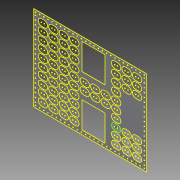
# Autodesk Inventor part: baseplate archive
Saved by Autodesk Inventor 2014 SP1 (Build 180222100, 222)
## iProperties
Created: 2014-01-05
Part Number: baseplate archive
Material: Aluminum 6061
Document SubType Name: Sheet Metal
Designer: Arpan
Density: 2.71 g/cm^3
Sheet Metal Rule: Default
Appearance: Aluminum - Flat
Mass: 756.379 g
Surface Area: 3765.41 cm^2
Volume: 279.107 cm^3
Author: Arpan
Autodesk Inventor part; units mm, degrees
(part 1 of 2)
ref_plane "YZ Plane" through (0, 0, 0) normal (1, 0, 0) x (0, 1, 0)
ref_plane "XZ Plane" through (0, 0, 0) normal (0, 1, 0) x (-1, 0, 0)
ref_plane "XY Plane" through (0, 0, 0) normal (0, 0, 1) x (1, 0, 0)
sketch "Sketch1" plane through (0, 0, 0) normal (0, 0, 1) x (1, 0, 0)
  line L0 (0, 0) -> (-685.8, 0)
  line L1 (-685.8, 0) -> (-685.8, 516.255)
  line L2 (-685.8, 516.255) -> (0, 516.255)
  line L3 (0, 516.255) -> (0, 0)
  dimension "d0" = 685.8
  dimension "d1" = 516.255
  measures "d0" distance of L1.end L2.end
  measures "d1" distance of L2.end L0.start
extrude "Plate1" add sketch "Sketch1" along normal blind 1.5875
sketch "Sketch4" plane through (0, 0, 1.5875) normal (0, 0, 1) x (1, 0, 0)
  circle A0 centre (-673.1, 503.555) radius 2.0828 projected
  circle A1 centre (-673.1, 12.7) radius 2.0828 projected
extrude "Cut3" cut sketch "Sketch4" against normal blind 1.5875
pattern_linear "Rectangular Pattern2" count 27 spacing 25.4 along (1, 0, 0) of "Cut3"
sketch "Sketch5" plane through (0, 0, 1.5875) normal (0, 0, 1) x (1, 0, 0)
  line L0 (-685.8, 516.255) -> (0, 516.255)
  line L1 (0, 516.255) -> (0, 0)
  line L2 (0, 0) -> (-685.8, 0)
  line L3 (-685.8, 0) -> (-685.8, 516.255)
  line L4 (-25.4, 490.855) -> (-660.4, 490.855)
  line L5 (-660.4, 490.855) -> (-660.4, 25.4)
  line L6 (-660.4, 25.4) -> (-25.4, 25.4)
  line L7 (-25.4, 25.4) -> (-25.4, 490.855)
  line L8 (-660.4, 490.855) -> (-596.9, 490.855)
  line L9 (-596.9, 490.855) -> (-596.9, 444.3095)
  line L10 (-596.9, 444.3095) -> (-660.4, 444.3095)
  line L11 (-660.4, 467.5822) -> (-596.9, 467.5822) construction
  line L12 (-637.1273, 444.3095) -> (-620.1728, 444.3095)
  line L13 (-620.1728, 490.855) -> (-637.1273, 490.855)
  arc A0 (-637.1273, 490.855) -> (-637.1273, 444.3095) centre (-637.1273, 467.5822) ccw
  arc A1 (-620.1728, 444.3095) -> (-620.1728, 490.855) centre (-620.1728, 467.5822) ccw
  line L14 (-620.1728, 487.68) -> (-637.1273, 487.68)
  arc A2 (-637.1273, 487.68) -> (-637.1273, 447.4845) centre (-637.1273, 467.5822) ccw
  line L15 (-637.1273, 447.4845) -> (-620.1728, 447.4845)
  arc A3 (-620.1728, 447.4845) -> (-620.1728, 487.68) centre (-620.1728, 467.5822) ccw
  point P0 (-412.75, 516.255)
  point P1 (-412.75, 0)
  point P2 (-273.05, 0)
  point P3 (-273.05, 516.255)
  point P4 (-628.65, 467.5822)
  dimension "d22" = 25.4
  dimension "d25" = 46.5455
  dimension "d28" = 3.175
  constraints: 34 end point, 10 point on circle, 6 parallel, 5 point on line, 4 centre point, 4 perpendicular, 4 tangent, 2 midpoint, 1 horizontal, 6 other
  measures "d22" distance between parallel lines of L0 L4
  measures "d25" distance of L8.end L9.end
  measures "d28" distance between parallel lines of L8 L14
extrude "Cut5" cut sketch "Sketch5" against normal blind 1.5875 contours A3 L15 A2 L14
pattern_linear "Rectangular Pattern3" count 10 spacing 46.5455 along (0, -1, 0) count 10 spacing 63.5 along (1, 0, 0) of "Cut5"
sketch "Sketch7" plane through (0, 0, 0) normal (0, 0, -1) x (-1, 0, 0)
  line L0 (256.1273, 75.1205) -> (239.1728, 75.1205)
  line L1 (402.7899, 184.15) -> (410.0101, 184.15)
  arc A0 (446.6273, 168.2115) -> (446.6273, 208.407) centre (446.6273, 188.3092) ccw
  arc A1 (429.6728, 208.407) -> (429.6728, 168.2115) centre (429.6728, 188.3092) ccw
  line L2 (412.75, 177.4677) -> (412.75, 152.6053)
  line L3 (273.05, 338.7873) -> (273.05, 363.6497)
  line L4 (283.0101, 332.105) -> (275.7899, 332.105)
  arc A2 (256.1273, 307.848) -> (256.1273, 348.0435) centre (256.1273, 327.9457) ccw
  arc A3 (239.1728, 348.0435) -> (239.1728, 307.848) centre (239.1728, 327.9457) ccw
  line L5 (429.6728, 188.3092) -> (446.6273, 188.3092) construction
  line L6 (429.6728, 168.2115) -> (446.6273, 168.2115)
  line L7 (446.6273, 208.407) -> (429.6728, 208.407)
  arc A4 (429.6728, 208.407) -> (429.6728, 168.2115) centre (429.6728, 188.3092) ccw
  arc A5 (446.6273, 168.2115) -> (446.6273, 208.407) centre (446.6273, 188.3092) ccw
  line L8 (366.1728, 168.2115) -> (383.1273, 168.2115)
  line L9 (383.1273, 208.407) -> (366.1728, 208.407)
  arc A6 (366.1728, 208.407) -> (366.1728, 168.2115) centre (366.1728, 188.3092) ccw
  arc A7 (383.1273, 168.2115) -> (383.1273, 208.407) centre (383.1273, 188.3092) ccw
  line L10 (302.6728, 168.2115) -> (319.6273, 168.2115)
  line L11 (319.6273, 208.407) -> (302.6728, 208.407)
  arc A8 (302.6728, 208.407) -> (302.6728, 168.2115) centre (302.6728, 188.3092) ccw
  arc A9 (319.6273, 168.2115) -> (319.6273, 208.407) centre (319.6273, 188.3092) ccw
  line L12 (239.1728, 168.2115) -> (256.1273, 168.2115)
  line L13 (256.1273, 208.407) -> (239.1728, 208.407)
  arc A10 (239.1728, 208.407) -> (239.1728, 168.2115) centre (239.1728, 188.3092) ccw
  arc A11 (256.1273, 168.2115) -> (256.1273, 208.407) centre (256.1273, 188.3092) ccw
  line L14 (429.6728, 121.666) -> (446.6273, 121.666)
  line L15 (446.6273, 161.8615) -> (429.6728, 161.8615)
  arc A12 (429.6728, 161.8615) -> (429.6728, 121.666) centre (429.6728, 141.7637) ccw
  arc A13 (446.6273, 121.666) -> (446.6273, 161.8615) centre (446.6273, 141.7637) ccw
  line L16 (366.1728, 121.666) -> (383.1273, 121.666)
  line L17 (383.1273, 161.8615) -> (366.1728, 161.8615)
  arc A14 (366.1728, 161.8615) -> (366.1728, 121.666) centre (366.1728, 141.7637) ccw
  arc A15 (383.1273, 121.666) -> (383.1273, 161.8615) centre (383.1273, 141.7637) ccw
  line L18 (302.6728, 121.666) -> (319.6273, 121.666)
  line L19 (319.6273, 161.8615) -> (302.6728, 161.8615)
  arc A16 (302.6728, 161.8615) -> (302.6728, 121.666) centre (302.6728, 141.7637) ccw
  arc A17 (319.6273, 121.666) -> (319.6273, 161.8615) centre (319.6273, 141.7637) ccw
  line L20 (239.1728, 121.666) -> (256.1273, 121.666)
  line L21 (256.1273, 161.8615) -> (239.1728, 161.8615)
  arc A18 (239.1728, 161.8615) -> (239.1728, 121.666) centre (239.1728, 141.7637) ccw
  arc A19 (256.1273, 121.666) -> (256.1273, 161.8615) centre (256.1273, 141.7637) ccw
  line L22 (429.6728, 75.1205) -> (446.6273, 75.1205)
  line L23 (446.6273, 115.316) -> (429.6728, 115.316)
  arc A20 (429.6728, 115.316) -> (429.6728, 75.1205) centre (429.6728, 95.2182) ccw
  arc A21 (446.6273, 75.1205) -> (446.6273, 115.316) centre (446.6273, 95.2182) ccw
  line L24 (366.1728, 75.1205) -> (383.1273, 75.1205)
  line L25 (383.1273, 115.316) -> (366.1728, 115.316)
  arc A22 (366.1728, 115.316) -> (366.1728, 75.1205) centre (366.1728, 95.2182) ccw
  arc A23 (383.1273, 75.1205) -> (383.1273, 115.316) centre (383.1273, 95.2182) ccw
  line L26 (302.6728, 75.1205) -> (319.6273, 75.1205)
  line L27 (319.6273, 115.316) -> (302.6728, 115.316)
  arc A24 (302.6728, 115.316) -> (302.6728, 75.1205) centre (302.6728, 95.2182) ccw
  arc A25 (319.6273, 75.1205) -> (319.6273, 115.316) centre (319.6273, 95.2182) ccw
  line L28 (239.1728, 75.1205) -> (256.1273, 75.1205)
  line L29 (256.1273, 115.316) -> (239.1728, 115.316)
  arc A26 (239.1728, 115.316) -> (239.1728, 75.1205) centre (239.1728, 95.2182) ccw
  arc A27 (256.1273, 75.1205) -> (256.1273, 115.316) centre (256.1273, 95.2182) ccw
  line L30 (429.6728, 28.575) -> (446.6273, 28.575)
  line L31 (446.6273, 68.7705) -> (429.6728, 68.7705)
  arc A28 (429.6728, 68.7705) -> (429.6728, 28.575) centre (429.6728, 48.6727) ccw
  arc A29 (446.6273, 28.575) -> (446.6273, 68.7705) centre (446.6273, 48.6727) ccw
  line L32 (366.1728, 28.575) -> (383.1273, 28.575)
  line L33 (383.1273, 68.7705) -> (366.1728, 68.7705)
  arc A30 (366.1728, 68.7705) -> (366.1728, 28.575) centre (366.1728, 48.6727) ccw
  arc A31 (383.1273, 28.575) -> (383.1273, 68.7705) centre (383.1273, 48.6727) ccw
  line L34 (302.6728, 28.575) -> (319.6273, 28.575)
  line L35 (319.6273, 68.7705) -> (302.6728, 68.7705)
  arc A32 (302.6728, 68.7705) -> (302.6728, 28.575) centre (302.6728, 48.6727) ccw
  arc A33 (319.6273, 28.575) -> (319.6273, 68.7705) centre (319.6273, 48.6727) ccw
  line L36 (239.1728, 28.575) -> (256.1273, 28.575)
  line L37 (256.1273, 68.7705) -> (239.1728, 68.7705)
  arc A34 (239.1728, 68.7705) -> (239.1728, 28.575) centre (239.1728, 48.6727) ccw
  arc A35 (256.1273, 28.575) -> (256.1273, 68.7705) centre (256.1273, 48.6727) ccw
  line L38 (239.1728, 327.9457) -> (256.1273, 327.9457) construction
  line L39 (239.1728, 307.848) -> (256.1273, 307.848)
  line L40 (256.1273, 348.0435) -> (239.1728, 348.0435)
  arc A36 (239.1728, 348.0435) -> (239.1728, 307.848) centre (239.1728, 327.9457) ccw
  arc A37 (256.1273, 307.848) -> (256.1273, 348.0435) centre (256.1273, 327.9457) ccw
  line L41 (239.1728, 354.3935) -> (256.1273, 354.3935)
  line L42 (256.1273, 394.589) -> (239.1728, 394.589)
  arc A38 (239.1728, 394.589) -> (239.1728, 354.3935) centre (239.1728, 374.4912) ccw
  arc A39 (256.1273, 354.3935) -> (256.1273, 394.589) centre (256.1273, 374.4912) ccw
  line L43 (239.1728, 400.939) -> (256.1273, 400.939)
  line L44 (256.1273, 441.1345) -> (239.1728, 441.1345)
  arc A40 (239.1728, 441.1345) -> (239.1728, 400.939) centre (239.1728, 421.0367) ccw
  arc A41 (256.1273, 400.939) -> (256.1273, 441.1345) centre (256.1273, 421.0367) ccw
  line L45 (239.1728, 447.4845) -> (256.1273, 447.4845)
  line L46 (256.1273, 487.68) -> (239.1728, 487.68)
  arc A42 (239.1728, 487.68) -> (239.1728, 447.4845) centre (239.1728, 467.5822) ccw
  arc A43 (256.1273, 447.4845) -> (256.1273, 487.68) centre (256.1273, 467.5822) ccw
  line L47 (302.6728, 307.848) -> (319.6273, 307.848)
  line L48 (319.6273, 348.0435) -> (302.6728, 348.0435)
  arc A44 (302.6728, 348.0435) -> (302.6728, 307.848) centre (302.6728, 327.9457) ccw
  arc A45 (319.6273, 307.848) -> (319.6273, 348.0435) centre (319.6273, 327.9457) ccw
  line L49 (302.6728, 354.3935) -> (319.6273, 354.3935)
  line L50 (319.6273, 394.589) -> (302.6728, 394.589)
  arc A46 (302.6728, 394.589) -> (302.6728, 354.3935) centre (302.6728, 374.4912) ccw
  arc A47 (319.6273, 354.3935) -> (319.6273, 394.589) centre (319.6273, 374.4912) ccw
  line L51 (302.6728, 400.939) -> (319.6273, 400.939)
  line L52 (319.6273, 441.1345) -> (302.6728, 441.1345)
  arc A48 (302.6728, 441.1345) -> (302.6728, 400.939) centre (302.6728, 421.0367) ccw
  arc A49 (319.6273, 400.939) -> (319.6273, 441.1345) centre (319.6273, 421.0367) ccw
  line L53 (302.6728, 447.4845) -> (319.6273, 447.4845)
  line L54 (319.6273, 487.68) -> (302.6728, 487.68)
  arc A50 (302.6728, 487.68) -> (302.6728, 447.4845) centre (302.6728, 467.5822) ccw
  arc A51 (319.6273, 447.4845) -> (319.6273, 487.68) centre (319.6273, 467.5822) ccw
  line L55 (366.1728, 307.848) -> (383.1273, 307.848)
  line L56 (383.1273, 348.0435) -> (366.1728, 348.0435)
  arc A52 (366.1728, 348.0435) -> (366.1728, 307.848) centre (366.1728, 327.9457) ccw
  arc A53 (383.1273, 307.848) -> (383.1273, 348.0435) centre (383.1273, 327.9457) ccw
  line L57 (366.1728, 354.3935) -> (383.1273, 354.3935)
  line L58 (383.1273, 394.589) -> (366.1728, 394.589)
  arc A54 (366.1728, 394.589) -> (366.1728, 354.3935) centre (366.1728, 374.4912) ccw
  arc A55 (383.1273, 354.3935) -> (383.1273, 394.589) centre (383.1273, 374.4912) ccw
  line L59 (366.1728, 400.939) -> (383.1273, 400.939)
  line L60 (383.1273, 441.1345) -> (366.1728, 441.1345)
  arc A56 (366.1728, 441.1345) -> (366.1728, 400.939) centre (366.1728, 421.0367) ccw
  arc A57 (383.1273, 400.939) -> (383.1273, 441.1345) centre (383.1273, 421.0367) ccw
  line L61 (366.1728, 447.4845) -> (383.1273, 447.4845)
  line L62 (383.1273, 487.68) -> (366.1728, 487.68)
  arc A58 (366.1728, 487.68) -> (366.1728, 447.4845) centre (366.1728, 467.5822) ccw
  arc A59 (383.1273, 447.4845) -> (383.1273, 487.68) centre (383.1273, 467.5822) ccw
  line L63 (429.6728, 307.848) -> (446.6273, 307.848)
  line L64 (446.6273, 348.0435) -> (429.6728, 348.0435)
  arc A60 (429.6728, 348.0435) -> (429.6728, 307.848) centre (429.6728, 327.9457) ccw
  arc A61 (446.6273, 307.848) -> (446.6273, 348.0435) centre (446.6273, 327.9457) ccw
  line L65 (429.6728, 354.3935) -> (446.6273, 354.3935)
  line L66 (446.6273, 394.589) -> (429.6728, 394.589)
  arc A62 (429.6728, 394.589) -> (429.6728, 354.3935) centre (429.6728, 374.4912) ccw
  arc A63 (446.6273, 354.3935) -> (446.6273, 394.589) centre (446.6273, 374.4912) ccw
  line L67 (429.6728, 400.939) -> (446.6273, 400.939)
  line L68 (446.6273, 441.1345) -> (429.6728, 441.1345)
  arc A64 (429.6728, 441.1345) -> (429.6728, 400.939) centre (429.6728, 421.0367) ccw
  arc A65 (446.6273, 400.939) -> (446.6273, 441.1345) centre (446.6273, 421.0367) ccw
  line L69 (429.6728, 447.4845) -> (446.6273, 447.4845)
  line L70 (446.6273, 487.68) -> (429.6728, 487.68)
  arc A66 (429.6728, 487.68) -> (429.6728, 447.4845) centre (429.6728, 467.5822) ccw
  arc A67 (446.6273, 447.4845) -> (446.6273, 487.68) centre (446.6273, 467.5822) ccw
  point P0 (438.15, 188.3092)
  point P1 (247.65, 327.9457)
  dimension "d46" = 63.5
  dimension "d49" = 46.5455
  dimension "d54" = 46.5455
  dimension "d57" = 63.5
  measures "d46" distance of L6.start L8.start
  measures "d49" distance of L6.start L14.start
  measures "d54" distance of L40.start L42.start
  measures "d57" distance of L40.start L48.start
sheet face with bend "Face2" sketch "Sketch7" thickness 1.5875 toward (0, 0, 1) bend radius 1.5875 relief tear relief width 1.5875 relief depth 0.7937
bend "Bend1"
sketch "Sketch2" plane through (0, 0, 1.5875) normal (0, 0, 1) x (1, 0, 0)
  line L0 (0, 0) -> (-685.8, 0) projected
  line L1 (-685.8, 516.255) -> (0, 516.255) projected
  line L2 (-342.9, 516.255) -> (-392.43, 516.255)
  line L3 (-392.43, 516.255) -> (-392.43, 332.105)
  line L4 (-392.43, 332.105) -> (-252.73, 332.105)
  line L5 (-252.73, 332.105) -> (-252.73, 516.255)
  line L6 (-392.43, 0) -> (-392.43, 184.15)
  line L7 (-392.43, 184.15) -> (-252.73, 184.15)
  line L8 (-252.73, 184.15) -> (-252.73, 0)
  line L9 (-392.43, 0) -> (-392.43, 25.4)
  line L10 (-392.43, 25.4) -> (-252.73, 25.4)
  line L11 (-252.73, 516.255) -> (-252.73, 490.855)
  line L12 (-252.73, 490.855) -> (-392.43, 490.855)
  line L13 (-685.8, 0) -> (-685.8, 516.255) projected
  dimension "d4" = 184.15
  dimension "d5" = 139.7
  dimension "d6" = 184.15
  dimension "d23" = 25.4
  dimension "d24" = 25.4
  dimension "d78" = 293.37
  dimension "d79" = 139.7
  dimension "d80" = 293.37
  constraints: 22 end point, 8 point on line, 6 perpendicular, 2 parallel, 1 midpoint
  measures "d4" distance of L2.end L3.end
  measures "d5" distance of L3.end L4.end
  measures "d6" distance of L6.start L6.end
  measures "d23" distance of L6.start L9.end
  measures "d24" distance of L5.end L11.end
  measures "d78" distance between parallel lines of L13 L6
  measures "d79" distance between parallel lines of L8 L6
  measures "d80" distance between parallel lines of L13 L3
extrude "Cut6" cut sketch "Sketch2" against normal blind 1.5875 contours L10 L6 L7 L8 | L12 L5 L4 L3
sketch "Sketch8" plane through (0, 0, 0) normal (0, 0, -1) x (-1, 0, 0)
  line L0 (252.73, 490.855) -> (392.43, 490.855)
  arc A0 (65.6273, 168.2115) -> (65.6273, 208.407) centre (65.6273, 188.3092) ccw
  line L1 (65.6273, 168.2115) -> (48.6728, 168.2115)
  arc A1 (48.6728, 208.407) -> (48.6728, 168.2115) centre (48.6728, 188.3092) ccw
  line L2 (48.6728, 208.407) -> (65.6273, 208.407)
  line L3 (48.6728, 188.3092) -> (65.6273, 188.3092) construction
  line L4 (48.6728, 168.2115) -> (65.6273, 168.2115)
  line L5 (65.6273, 208.407) -> (48.6728, 208.407)
  arc A2 (48.6728, 208.407) -> (48.6728, 168.2115) centre (48.6728, 188.3092) ccw
  arc A3 (65.6273, 168.2115) -> (65.6273, 208.407) centre (65.6273, 188.3092) ccw
  point P0 (57.15, 188.3092)
sheet face with bend "Face3" sketch "Sketch8" thickness 1.5875 toward (0, 0, 1) bend radius 1.5875 relief tear relief width 1.5875 relief depth 0.7937
bend "Bend2"
pattern_linear "Rectangular Pattern4" count 2 spacing 63.5 along (-1, 0, 0) count 4 spacing 46.5455 along (0, 1, 0) of "Face3"
sketch "Sketch10" plane through (0, 0, 0) normal (0, 0, -1) x (-1, 0, 0)
  line L0 (252.73, 490.855) -> (392.43, 490.855) projected
  line L1 (392.43, 490.855) -> (392.43, 332.105) projected
  arc A0 (510.1273, 447.4845) -> (510.1273, 487.68) centre (510.1273, 467.5822) ccw projected
  arc A1 (493.1728, 487.68) -> (493.1728, 447.4845) centre (493.1728, 467.5822) ccw projected
  line L2 (685.8, 516.255) -> (0, 516.255) projected
  line L3 (444.5, 487.68) -> (427.1544, 487.68)
  line L4 (429.6728, 467.5822) -> (446.6273, 467.5822) construction
  line L5 (429.6728, 447.4845) -> (446.6273, 447.4845)
  line L6 (446.6273, 487.68) -> (429.6728, 487.68)
  arc A2 (429.6728, 487.68) -> (429.6728, 447.4845) centre (429.6728, 467.5822) ccw
  arc A3 (446.6273, 447.4845) -> (446.6273, 487.68) centre (446.6273, 467.5822) ccw
  line L7 (429.6728, 400.939) -> (446.6273, 400.939)
  line L8 (446.6273, 441.1345) -> (429.6728, 441.1345)
  arc A4 (429.6728, 441.1345) -> (429.6728, 400.939) centre (429.6728, 421.0367) ccw
  arc A5 (446.6273, 400.939) -> (446.6273, 441.1345) centre (446.6273, 421.0367) ccw
  line L9 (429.6728, 354.3935) -> (446.6273, 354.3935)
  line L10 (446.6273, 394.589) -> (429.6728, 394.589)
  arc A6 (429.6728, 394.589) -> (429.6728, 354.3935) centre (429.6728, 374.4912) ccw
  arc A7 (446.6273, 354.3935) -> (446.6273, 394.589) centre (446.6273, 374.4912) ccw
  line L11 (429.6728, 307.848) -> (446.6273, 307.848)
  line L12 (446.6273, 348.0435) -> (429.6728, 348.0435)
  arc A8 (429.6728, 348.0435) -> (429.6728, 307.848) centre (429.6728, 327.9457) ccw
  arc A9 (446.6273, 307.848) -> (446.6273, 348.0435) centre (446.6273, 327.9457) ccw
  line L13 (429.6728, 261.3025) -> (446.6273, 261.3025)
  line L14 (446.6273, 301.498) -> (429.6728, 301.498)
  arc A10 (429.6728, 301.498) -> (429.6728, 261.3025) centre (429.6728, 281.4002) ccw
  arc A11 (446.6273, 261.3025) -> (446.6273, 301.498) centre (446.6273, 281.4002) ccw
  line L15 (429.6728, 214.757) -> (446.6273, 214.757)
  line L16 (446.6273, 254.9525) -> (429.6728, 254.9525)
  arc A12 (429.6728, 254.9525) -> (429.6728, 214.757) centre (429.6728, 234.8547) ccw
  arc A13 (446.6273, 214.757) -> (446.6273, 254.9525) centre (446.6273, 234.8547) ccw
  line L17 (429.6728, 168.2115) -> (446.6273, 168.2115)
  line L18 (446.6273, 208.407) -> (429.6728, 208.407)
  arc A14 (429.6728, 208.407) -> (429.6728, 168.2115) centre (429.6728, 188.3092) ccw
  arc A15 (446.6273, 168.2115) -> (446.6273, 208.407) centre (446.6273, 188.3092) ccw
  line L19 (429.6728, 121.666) -> (446.6273, 121.666)
  line L20 (446.6273, 161.8615) -> (429.6728, 161.8615)
  arc A16 (429.6728, 161.8615) -> (429.6728, 121.666) centre (429.6728, 141.7637) ccw
  arc A17 (446.6273, 121.666) -> (446.6273, 161.8615) centre (446.6273, 141.7637) ccw
  line L21 (429.6728, 75.1205) -> (446.6273, 75.1205)
  line L22 (446.6273, 115.316) -> (429.6728, 115.316)
  arc A18 (429.6728, 115.316) -> (429.6728, 75.1205) centre (429.6728, 95.2182) ccw
  arc A19 (446.6273, 75.1205) -> (446.6273, 115.316) centre (446.6273, 95.2182) ccw
  line L23 (429.6728, 28.575) -> (446.6273, 28.575)
  line L24 (446.6273, 68.7705) -> (429.6728, 68.7705)
  arc A20 (429.6728, 68.7705) -> (429.6728, 28.575) centre (429.6728, 48.6727) ccw
  arc A21 (446.6273, 28.575) -> (446.6273, 68.7705) centre (446.6273, 48.6727) ccw
  point P0 (438.15, 467.5822)
  point P1 (444.5, 441.1345)
  point P2 (444.5, 394.589)
  point P3 (444.5, 348.0435)
  point P4 (444.5, 301.498)
  point P5 (444.5, 254.9525)
  point P6 (444.5, 208.407)
  point P7 (444.5, 161.8615)
  point P8 (444.5, 115.316)
  point P9 (444.5, 68.7705)
  dimension "d83" = 63.5
  dimension "d90" = 46.5455
  constraints: 46 end point, 40 point on circle, 20 centre point, 4 tangent, 2 parallel, 1 horizontal, 1 midpoint, 1 vertical, 101 other
  measures "d83" distance of A1.centre L4.start
  measures "d90" distance of L5.start L7.start
extrude "Cut7" cut sketch "Sketch10" against normal blind 1.5875 contours L6 A3 L5 A2 L3 | A4 L8 A5 L7 | A6 L10 A7 L9 | A8 L12 A9 L11 | A14 L18 A15 L17 | A16 L20 A17 L19 | A18 L22 A19 L21 | A20 L24 A21 L23
sketch "Sketch12" plane through (0, 0, 1.5875) normal (0, 0, 1) x (1, 0, 0)
  arc A0 (-673.1762, 31.5962) -> (-673.1762, 27.4588) centre (-673.1, 29.5275) ccw projected
  arc A1 (-673.0238, 27.4588) -> (-673.0238, 31.5962) centre (-673.1, 29.5275) ccw projected
  circle A2 centre (-673.1, 29.5275) radius 2.0701
  constraints: 1 centre point, 1 coincident, 1 concentric
extrude "Cut8" cut sketch "Sketch12" against normal blind 1.5875
pattern_linear "Rectangular Pattern5" count 19 spacing 25.4 along (0, 1, 0) count 2 spacing 660.4 along (1, 0, 0) of "Cut8"
sketch "Sketch13" plane through (0, 0, 1.5875) normal (0, 0, 1) x (1, 0, 0)
  circle A0 centre (-12.7, 486.7275) radius 2.0701 projected
  circle A1 centre (-12.7, 461.3275) radius 2.0701 projected
  circle A2 centre (-12.7, 435.9275) radius 2.0701 projected
  circle A3 centre (-12.7, 410.5275) radius 2.0701 projected
  circle A4 centre (-12.7, 385.1275) radius 2.0701 projected
  circle A5 centre (-12.7, 359.7275) radius 2.0701 projected
  circle A6 centre (-12.7, 334.3275) radius 2.0701 projected
  circle A7 centre (-12.7, 308.9275) radius 2.0701 projected
  circle A8 centre (-12.7, 283.5275) radius 2.0701 projected
  circle A9 centre (-12.7, 258.1275) radius 2.0701 projected
  circle A10 centre (-12.7, 232.7275) radius 2.0701 projected
  circle A11 centre (-12.7, 207.3275) radius 2.0701 projected
  circle A12 centre (-12.7, 181.9275) radius 2.0701 projected
  circle A13 centre (-12.7, 156.5275) radius 2.0701 projected
  circle A14 centre (-12.7, 131.1275) radius 2.0701 projected
  circle A15 centre (-12.7, 105.7275) radius 2.0701 projected
  circle A16 centre (-12.7, 80.3275) radius 2.0701 projected
  circle A17 centre (-12.7, 54.9275) radius 2.0701 projected
  circle A18 centre (-12.7, 29.5275) radius 2.0701 projected
  circle A19 centre (-673.1, 486.7275) radius 2.0701 projected
  circle A20 centre (-673.1, 461.3275) radius 2.0701 projected
  circle A21 centre (-673.1, 435.9275) radius 2.0701 projected
  circle A22 centre (-673.1, 410.5275) radius 2.0701 projected
  circle A23 centre (-673.1, 385.1275) radius 2.0701 projected
  circle A24 centre (-673.1, 359.7275) radius 2.0701 projected
  circle A25 centre (-673.1, 334.3275) radius 2.0701 projected
  circle A26 centre (-673.1, 308.9275) radius 2.0701 projected
  circle A27 centre (-673.1, 283.5275) radius 2.0701 projected
  circle A28 centre (-673.1, 258.1275) radius 2.0701 projected
  circle A29 centre (-673.1, 232.7275) radius 2.0701 projected
  circle A30 centre (-673.1, 207.3275) radius 2.0701 projected
  circle A31 centre (-673.1, 181.9275) radius 2.0701 projected
  circle A32 centre (-673.1, 156.5275) radius 2.0701 projected
  circle A33 centre (-673.1, 131.1275) radius 2.0701 projected
  circle A34 centre (-673.1, 105.7275) radius 2.0701 projected
  circle A35 centre (-673.1, 80.3275) radius 2.0701 projected
  circle A36 centre (-673.1, 54.9275) radius 2.0701 projected
  circle A37 centre (-673.1, 29.5275) radius 2.0701 projected
  arc A38 (-446.6273, 115.316) -> (-446.6273, 75.1205) centre (-446.6273, 95.2182) ccw projected
  line L0 (-446.6273, 115.316) -> (-429.6728, 115.316) projected
  arc A39 (-429.6728, 75.1205) -> (-429.6728, 115.316) centre (-429.6728, 95.2182) ccw projected
  line L1 (-429.6728, 75.1205) -> (-446.6273, 75.1205) projected
  arc A40 (-446.6273, 208.407) -> (-446.6273, 168.2115) centre (-446.6273, 188.3092) ccw projected
  line L2 (-446.6273, 208.407) -> (-429.6728, 208.407) projected
  arc A41 (-429.6728, 168.2115) -> (-429.6728, 208.407) centre (-429.6728, 188.3092) ccw projected
  line L3 (-429.6728, 168.2115) -> (-446.6273, 168.2115) projected
  arc A42 (-446.6273, 394.589) -> (-446.6273, 354.3935) centre (-446.6273, 374.4912) ccw projected
  line L4 (-446.6273, 394.589) -> (-429.6728, 394.589) projected
  arc A43 (-429.6728, 354.3935) -> (-429.6728, 394.589) centre (-429.6728, 374.4912) ccw projected
  line L5 (-429.6728, 354.3935) -> (-446.6273, 354.3935) projected
  arc A44 (-446.6273, 487.68) -> (-446.6273, 447.4845) centre (-446.6273, 467.5822) ccw projected
  line L6 (-446.6273, 487.68) -> (-429.6728, 487.68) projected
  arc A45 (-429.6728, 447.4845) -> (-429.6728, 487.68) centre (-429.6728, 467.5822) ccw projected
  line L7 (-429.6728, 447.4845) -> (-446.6273, 447.4845) projected
  arc A46 (-446.6273, 441.1345) -> (-446.6273, 400.939) centre (-446.6273, 421.0367) ccw projected
  line L8 (-446.6273, 441.1345) -> (-429.6728, 441.1345) projected
  arc A47 (-429.6728, 400.939) -> (-429.6728, 441.1345) centre (-429.6728, 421.0367) ccw projected
  line L9 (-429.6728, 400.939) -> (-446.6273, 400.939) projected
  arc A48 (-446.6273, 348.0435) -> (-446.6273, 307.848) centre (-446.6273, 327.9457) ccw projected
  line L10 (-446.6273, 348.0435) -> (-429.6728, 348.0435) projected
  arc A49 (-429.6728, 307.848) -> (-429.6728, 348.0435) centre (-429.6728, 327.9457) ccw projected
  line L11 (-429.6728, 307.848) -> (-446.6273, 307.848) projected
  arc A50 (-446.6273, 161.8615) -> (-446.6273, 121.666) centre (-446.6273, 141.7637) ccw projected
  line L12 (-446.6273, 161.8615) -> (-429.6728, 161.8615) projected
  arc A51 (-429.6728, 121.666) -> (-429.6728, 161.8615) centre (-429.6728, 141.7637) ccw projected
  line L13 (-429.6728, 121.666) -> (-446.6273, 121.666) projected
  arc A52 (-446.6273, 68.7705) -> (-446.6273, 28.575) centre (-446.6273, 48.6727) ccw projected
  line L14 (-446.6273, 68.7705) -> (-429.6728, 68.7705) projected
  arc A53 (-429.6728, 28.575) -> (-429.6728, 68.7705) centre (-429.6728, 48.6727) ccw projected
  line L15 (-429.6728, 28.575) -> (-446.6273, 28.575) projected
  line L16 (-252.73, 490.855) -> (-252.73, 332.105) projected
  line L17 (-252.73, 332.105) -> (-392.43, 332.105) projected
  line L18 (-392.43, 332.105) -> (-392.43, 490.855) projected
  line L19 (-392.43, 490.855) -> (-252.73, 490.855) projected
  line L20 (-252.73, 25.4) -> (-392.43, 25.4) projected
  line L21 (-392.43, 25.4) -> (-392.43, 184.15) projected
  line L22 (-392.43, 184.15) -> (-252.73, 184.15) projected
  line L23 (-252.73, 184.15) -> (-252.73, 25.4) projected
  arc A54 (-65.6272, 68.7705) -> (-65.6272, 28.575) centre (-65.6272, 48.6727) ccw projected
  line L24 (-65.6272, 68.7705) -> (-48.6728, 68.7705) projected
  arc A55 (-48.6728, 28.575) -> (-48.6728, 68.7705) centre (-48.6728, 48.6727) ccw projected
  line L25 (-48.6728, 28.575) -> (-65.6272, 28.575) projected
  arc A56 (-65.6273, 115.316) -> (-65.6273, 75.1205) centre (-65.6273, 95.2182) ccw projected
  line L26 (-65.6273, 115.316) -> (-48.6728, 115.316) projected
  arc A57 (-48.6728, 75.1205) -> (-48.6728, 115.316) centre (-48.6728, 95.2182) ccw projected
  line L27 (-48.6728, 75.1205) -> (-65.6273, 75.1205) projected
  arc A58 (-65.6273, 161.8615) -> (-65.6273, 121.666) centre (-65.6273, 141.7637) ccw projected
  line L28 (-65.6273, 161.8615) -> (-48.6728, 161.8615) projected
  arc A59 (-48.6728, 121.666) -> (-48.6728, 161.8615) centre (-48.6728, 141.7637) ccw projected
  line L29 (-48.6728, 121.666) -> (-65.6273, 121.666) projected
  arc A60 (-65.6273, 394.589) -> (-65.6273, 354.3935) centre (-65.6273, 374.4912) ccw projected
  line L30 (-65.6273, 394.589) -> (-48.6728, 394.589) projected
  arc A61 (-48.6728, 354.3935) -> (-48.6728, 394.589) centre (-48.6728, 374.4912) ccw projected
  line L31 (-48.6728, 354.3935) -> (-65.6273, 354.3935) projected
  arc A62 (-65.6273, 441.1345) -> (-65.6273, 400.939) centre (-65.6273, 421.0367) ccw projected
  line L32 (-65.6273, 441.1345) -> (-48.6728, 441.1345) projected
  arc A63 (-48.6728, 400.939) -> (-48.6728, 441.1345) centre (-48.6728, 421.0367) ccw projected
  line L33 (-48.6728, 400.939) -> (-65.6273, 400.939) projected
  arc A64 (-65.6273, 487.68) -> (-65.6273, 447.4845) centre (-65.6273, 467.5822) ccw projected
  line L34 (-65.6273, 487.68) -> (-48.6728, 487.68) projected
  arc A65 (-48.6728, 447.4845) -> (-48.6728, 487.68) centre (-48.6728, 467.5822) ccw projected
  line L35 (-48.6728, 447.4845) -> (-65.6273, 447.4845) projected
  arc A66 (-129.1272, 68.7705) -> (-129.1272, 28.575) centre (-129.1272, 48.6727) ccw projected
  line L36 (-129.1272, 68.7705) -> (-112.1728, 68.7705) projected
  arc A67 (-112.1728, 28.575) -> (-112.1728, 68.7705) centre (-112.1728, 48.6727) ccw projected
  line L37 (-112.1728, 28.575) -> (-129.1272, 28.575) projected
  arc A68 (-129.1273, 115.316) -> (-129.1273, 75.1205) centre (-129.1273, 95.2182) ccw projected
  line L38 (-129.1273, 115.316) -> (-112.1728, 115.316) projected
  arc A69 (-112.1728, 75.1205) -> (-112.1728, 115.316) centre (-112.1728, 95.2182) ccw projected
  line L39 (-112.1728, 75.1205) -> (-129.1273, 75.1205) projected
  arc A70 (-129.1273, 161.8615) -> (-129.1273, 121.666) centre (-129.1273, 141.7637) ccw projected
  line L40 (-129.1273, 161.8615) -> (-112.1728, 161.8615) projected
  arc A71 (-112.1728, 121.666) -> (-112.1728, 161.8615) centre (-112.1728, 141.7637) ccw projected
  line L41 (-112.1728, 121.666) -> (-129.1273, 121.666) projected
  arc A72 (-129.1273, 394.589) -> (-129.1273, 354.3935) centre (-129.1273, 374.4912) ccw projected
  line L42 (-129.1273, 394.589) -> (-112.1728, 394.589) projected
  arc A73 (-112.1728, 354.3935) -> (-112.1728, 394.589) centre (-112.1728, 374.4912) ccw projected
  line L43 (-112.1728, 354.3935) -> (-129.1273, 354.3935) projected
  arc A74 (-129.1273, 441.1345) -> (-129.1273, 400.939) centre (-129.1273, 421.0367) ccw projected
  line L44 (-129.1273, 441.1345) -> (-112.1728, 441.1345) projected
  arc A75 (-112.1728, 400.939) -> (-112.1728, 441.1345) centre (-112.1728, 421.0367) ccw projected
  line L45 (-112.1728, 400.939) -> (-129.1273, 400.939) projected
  arc A76 (-129.1273, 487.68) -> (-129.1273, 447.4845) centre (-129.1273, 467.5822) ccw projected
  line L46 (-129.1273, 487.68) -> (-112.1728, 487.68) projected
  arc A77 (-112.1728, 447.4845) -> (-112.1728, 487.68) centre (-112.1728, 467.5822) ccw projected
  line L47 (-112.1728, 447.4845) -> (-129.1273, 447.4845) projected
  arc A78 (-192.6272, 68.7705) -> (-192.6272, 28.575) centre (-192.6272, 48.6727) ccw projected
  line L48 (-192.6272, 68.7705) -> (-175.6728, 68.7705) projected
  arc A79 (-175.6728, 28.575) -> (-175.6728, 68.7705) centre (-175.6728, 48.6727) ccw projected
  line L49 (-175.6728, 28.575) -> (-192.6272, 28.575) projected
  arc A80 (-192.6273, 115.316) -> (-192.6273, 75.1205) centre (-192.6273, 95.2182) ccw projected
  line L50 (-192.6273, 115.316) -> (-175.6728, 115.316) projected
  arc A81 (-175.6728, 75.1205) -> (-175.6728, 115.316) centre (-175.6728, 95.2182) ccw projected
  line L51 (-175.6728, 75.1205) -> (-192.6273, 75.1205) projected
  arc A82 (-192.6273, 161.8615) -> (-192.6273, 121.666) centre (-192.6273, 141.7637) ccw projected
  line L52 (-192.6273, 161.8615) -> (-175.6728, 161.8615) projected
  arc A83 (-175.6728, 121.666) -> (-175.6728, 161.8615) centre (-175.6728, 141.7637) ccw projected
  line L53 (-175.6728, 121.666) -> (-192.6273, 121.666) projected
  arc A84 (-192.6273, 208.407) -> (-192.6273, 168.2115) centre (-192.6273, 188.3092) ccw projected
  line L54 (-192.6273, 208.407) -> (-175.6728, 208.407) projected
  arc A85 (-175.6728, 168.2115) -> (-175.6728, 208.407) centre (-175.6728, 188.3092) ccw projected
  line L55 (-175.6728, 168.2115) -> (-192.6273, 168.2115) projected
  arc A86 (-192.6273, 254.9525) -> (-192.6273, 214.757) centre (-192.6273, 234.8547) ccw projected
  line L56 (-192.6273, 254.9525) -> (-175.6728, 254.9525) projected
  arc A87 (-175.6728, 214.757) -> (-175.6728, 254.9525) centre (-175.6728, 234.8547) ccw projected
  line L57 (-175.6728, 214.757) -> (-192.6273, 214.757) projected
  arc A88 (-192.6273, 301.498) -> (-192.6273, 261.3025) centre (-192.6273, 281.4002) ccw projected
  line L58 (-192.6273, 301.498) -> (-175.6728, 301.498) projected
  arc A89 (-175.6728, 261.3025) -> (-175.6728, 301.498) centre (-175.6728, 281.4002) ccw projected
  line L59 (-175.6728, 261.3025) -> (-192.6273, 261.3025) projected
  arc A90 (-192.6273, 348.0435) -> (-192.6273, 307.848) centre (-192.6273, 327.9457) ccw projected
  line L60 (-192.6273, 348.0435) -> (-175.6728, 348.0435) projected
  arc A91 (-175.6728, 307.848) -> (-175.6728, 348.0435) centre (-175.6728, 327.9457) ccw projected
  line L61 (-175.6728, 307.848) -> (-192.6273, 307.848) projected
  arc A92 (-192.6273, 394.589) -> (-192.6273, 354.3935) centre (-192.6273, 374.4912) ccw projected
  line L62 (-192.6273, 394.589) -> (-175.6728, 394.589) projected
  arc A93 (-175.6728, 354.3935) -> (-175.6728, 394.589) centre (-175.6728, 374.4912) ccw projected
  line L63 (-175.6728, 354.3935) -> (-192.6273, 354.3935) projected
  arc A94 (-192.6273, 441.1345) -> (-192.6273, 400.939) centre (-192.6273, 421.0367) ccw projected
  line L64 (-192.6273, 441.1345) -> (-175.6728, 441.1345) projected
  arc A95 (-175.6728, 400.939) -> (-175.6728, 441.1345) centre (-175.6728, 421.0367) ccw projected
  line L65 (-175.6728, 400.939) -> (-192.6273, 400.939) projected
  arc A96 (-192.6273, 487.68) -> (-192.6273, 447.4845) centre (-192.6273, 467.5822) ccw projected
  line L66 (-192.6273, 487.68) -> (-175.6728, 487.68) projected
  arc A97 (-175.6728, 447.4845) -> (-175.6728, 487.68) centre (-175.6728, 467.5822) ccw projected
  line L67 (-175.6728, 447.4845) -> (-192.6273, 447.4845) projected
  arc A98 (-256.1273, 254.9525) -> (-256.1273, 214.757) centre (-256.1273, 234.8547) ccw projected
  line L68 (-256.1273, 254.9525) -> (-239.1728, 254.9525) projected
  arc A99 (-239.1728, 214.757) -> (-239.1728, 254.9525) centre (-239.1728, 234.8547) ccw projected
  line L69 (-239.1728, 214.757) -> (-256.1273, 214.757) projected
  arc A100 (-256.1273, 301.498) -> (-256.1273, 261.3025) centre (-256.1273, 281.4002) ccw projected
  line L70 (-256.1273, 301.498) -> (-239.1728, 301.498) projected
  arc A101 (-239.1728, 261.3025) -> (-239.1728, 301.498) centre (-239.1728, 281.4002) ccw projected
  line L71 (-239.1728, 261.3025) -> (-256.1273, 261.3025) projected
  arc A102 (-319.6273, 254.9525) -> (-319.6273, 214.757) centre (-319.6273, 234.8547) ccw projected
  line L72 (-319.6273, 254.9525) -> (-302.6728, 254.9525) projected
  arc A103 (-302.6728, 214.757) -> (-302.6728, 254.9525) centre (-302.6728, 234.8547) ccw projected
  line L73 (-302.6728, 214.757) -> (-319.6273, 214.757) projected
  arc A104 (-319.6273, 301.498) -> (-319.6273, 261.3025) centre (-319.6273, 281.4002) ccw projected
  line L74 (-319.6273, 301.498) -> (-302.6728, 301.498) projected
  arc A105 (-302.6728, 261.3025) -> (-302.6728, 301.498) centre (-302.6728, 281.4002) ccw projected
  line L75 (-302.6728, 261.3025) -> (-319.6273, 261.3025) projected
  arc A106 (-383.1273, 254.9525) -> (-383.1273, 214.757) centre (-383.1273, 234.8547) ccw projected
  line L76 (-383.1273, 254.9525) -> (-366.1728, 254.9525) projected
  arc A107 (-366.1728, 214.757) -> (-366.1728, 254.9525) centre (-366.1728, 234.8547) ccw projected
  line L77 (-366.1728, 214.757) -> (-383.1273, 214.757) projected
  arc A108 (-383.1273, 301.498) -> (-383.1273, 261.3025) centre (-383.1273, 281.4002) ccw projected
  line L78 (-383.1273, 301.498) -> (-366.1728, 301.498) projected
  arc A109 (-366.1728, 261.3025) -> (-366.1728, 301.498) centre (-366.1728, 281.4002) ccw projected
  line L79 (-366.1728, 261.3025) -> (-383.1273, 261.3025) projected
  arc A110 (-446.6273, 254.9525) -> (-446.6273, 214.757) centre (-446.6273, 234.8547) ccw projected
  line L80 (-446.6273, 254.9525) -> (-429.6728, 254.9525) projected
  arc A111 (-429.6728, 214.757) -> (-429.6728, 254.9525) centre (-429.6728, 234.8547) ccw projected
  line L81 (-429.6728, 214.757) -> (-446.6273, 214.757) projected
  arc A112 (-446.6273, 301.498) -> (-446.6273, 261.3025) centre (-446.6273, 281.4002) ccw projected
  line L82 (-446.6273, 301.498) -> (-429.6728, 301.498) projected
  arc A113 (-429.6728, 261.3025) -> (-429.6728, 301.498) centre (-429.6728, 281.4002) ccw projected
  line L83 (-429.6728, 261.3025) -> (-446.6273, 261.3025) projected
  arc A114 (-510.1272, 68.7705) -> (-510.1272, 28.575) centre (-510.1272, 48.6727) ccw projected
  line L84 (-510.1272, 68.7705) -> (-493.1728, 68.7705) projected
  arc A115 (-493.1728, 28.575) -> (-493.1728, 68.7705) centre (-493.1728, 48.6727) ccw projected
  line L85 (-493.1728, 28.575) -> (-510.1272, 28.575) projected
  arc A116 (-510.1272, 115.316) -> (-510.1272, 75.1205) centre (-510.1272, 95.2182) ccw projected
  line L86 (-510.1272, 115.316) -> (-493.1728, 115.316) projected
  arc A117 (-493.1728, 75.1205) -> (-493.1728, 115.316) centre (-493.1728, 95.2182) ccw projected
  line L87 (-493.1728, 75.1205) -> (-510.1272, 75.1205) projected
  arc A118 (-510.1272, 161.8615) -> (-510.1272, 121.666) centre (-510.1272, 141.7637) ccw projected
  line L88 (-510.1272, 161.8615) -> (-493.1728, 161.8615) projected
  arc A119 (-493.1728, 121.666) -> (-493.1728, 161.8615) centre (-493.1728, 141.7637) ccw projected
  line L89 (-493.1728, 121.666) -> (-510.1272, 121.666) projected
  arc A120 (-510.1273, 208.407) -> (-510.1273, 168.2115) centre (-510.1273, 188.3092) ccw projected
  line L90 (-510.1273, 208.407) -> (-493.1728, 208.407) projected
  arc A121 (-493.1728, 168.2115) -> (-493.1728, 208.407) centre (-493.1728, 188.3092) ccw projected
  line L91 (-493.1728, 168.2115) -> (-510.1273, 168.2115) projected
  arc A122 (-510.1273, 254.9525) -> (-510.1273, 214.757) centre (-510.1273, 234.8547) ccw projected
  line L92 (-510.1273, 254.9525) -> (-493.1728, 254.9525) projected
  arc A123 (-493.1728, 214.757) -> (-493.1728, 254.9525) centre (-493.1728, 234.8547) ccw projected
  line L93 (-493.1728, 214.757) -> (-510.1273, 214.757) projected
  arc A124 (-510.1273, 301.498) -> (-510.1273, 261.3025) centre (-510.1273, 281.4002) ccw projected
  line L94 (-510.1273, 301.498) -> (-493.1728, 301.498) projected
  arc A125 (-493.1728, 261.3025) -> (-493.1728, 301.498) centre (-493.1728, 281.4002) ccw projected
  line L95 (-493.1728, 261.3025) -> (-510.1273, 261.3025) projected
  arc A126 (-510.1273, 348.0435) -> (-510.1273, 307.848) centre (-510.1273, 327.9457) ccw projected
  line L96 (-510.1273, 348.0435) -> (-493.1728, 348.0435) projected
  arc A127 (-493.1728, 307.848) -> (-493.1728, 348.0435) centre (-493.1728, 327.9457) ccw projected
  line L97 (-493.1728, 307.848) -> (-510.1273, 307.848) projected
  arc A128 (-510.1273, 394.589) -> (-510.1273, 354.3935) centre (-510.1273, 374.4912) ccw projected
  line L98 (-510.1273, 394.589) -> (-493.1728, 394.589) projected
  arc A129 (-493.1728, 354.3935) -> (-493.1728, 394.589) centre (-493.1728, 374.4912) ccw projected
  line L99 (-493.1728, 354.3935) -> (-510.1273, 354.3935) projected
  arc A130 (-510.1273, 441.1345) -> (-510.1273, 400.939) centre (-510.1273, 421.0367) ccw projected
  line L100 (-510.1273, 441.1345) -> (-493.1728, 441.1345) projected
  arc A131 (-493.1728, 400.939) -> (-493.1728, 441.1345) centre (-493.1728, 421.0367) ccw projected
  line L101 (-493.1728, 400.939) -> (-510.1273, 400.939) projected
  arc A132 (-510.1273, 487.68) -> (-510.1273, 447.4845) centre (-510.1273, 467.5822) ccw projected
  line L102 (-510.1273, 487.68) -> (-493.1728, 487.68) projected
  arc A133 (-493.1728, 447.4845) -> (-493.1728, 487.68) centre (-493.1728, 467.5822) ccw projected
  line L103 (-493.1728, 447.4845) -> (-510.1273, 447.4845) projected
  arc A134 (-573.6273, 68.7705) -> (-573.6273, 28.575) centre (-573.6273, 48.6727) ccw projected
  line L104 (-573.6273, 68.7705) -> (-556.6728, 68.7705) projected
  arc A135 (-556.6728, 28.575) -> (-556.6728, 68.7705) centre (-556.6728, 48.6727) ccw projected
  line L105 (-556.6728, 28.575) -> (-573.6273, 28.575) projected
  arc A136 (-573.6273, 115.316) -> (-573.6273, 75.1205) centre (-573.6273, 95.2182) ccw projected
  line L106 (-573.6273, 115.316) -> (-556.6728, 115.316) projected
  arc A137 (-556.6728, 75.1205) -> (-556.6728, 115.316) centre (-556.6728, 95.2182) ccw projected
  line L107 (-556.6728, 75.1205) -> (-573.6273, 75.1205) projected
  arc A138 (-573.6273, 161.8615) -> (-573.6273, 121.666) centre (-573.6273, 141.7637) ccw projected
  line L108 (-573.6273, 161.8615) -> (-556.6728, 161.8615) projected
  arc A139 (-556.6728, 121.666) -> (-556.6728, 161.8615) centre (-556.6728, 141.7637) ccw projected
  line L109 (-556.6728, 121.666) -> (-573.6273, 121.666) projected
  arc A140 (-573.6273, 208.407) -> (-573.6273, 168.2115) centre (-573.6273, 188.3092) ccw projected
  line L110 (-573.6273, 208.407) -> (-556.6728, 208.407) projected
  arc A141 (-556.6728, 168.2115) -> (-556.6728, 208.407) centre (-556.6728, 188.3092) ccw projected
  line L111 (-556.6728, 168.2115) -> (-573.6273, 168.2115) projected
  arc A142 (-573.6273, 254.9525) -> (-573.6273, 214.757) centre (-573.6273, 234.8547) ccw projected
  line L112 (-573.6273, 254.9525) -> (-556.6728, 254.9525) projected
  arc A143 (-556.6728, 214.757) -> (-556.6728, 254.9525) centre (-556.6728, 234.8547) ccw projected
  line L113 (-556.6728, 214.757) -> (-573.6273, 214.757) projected
  arc A144 (-573.6273, 301.498) -> (-573.6273, 261.3025) centre (-573.6273, 281.4002) ccw projected
  line L114 (-573.6273, 301.498) -> (-556.6728, 301.498) projected
  arc A145 (-556.6728, 261.3025) -> (-556.6728, 301.498) centre (-556.6728, 281.4002) ccw projected
  line L115 (-556.6728, 261.3025) -> (-573.6273, 261.3025) projected
  arc A146 (-573.6273, 348.0435) -> (-573.6273, 307.848) centre (-573.6273, 327.9457) ccw projected
  line L116 (-573.6273, 348.0435) -> (-556.6728, 348.0435) projected
  arc A147 (-556.6728, 307.848) -> (-556.6728, 348.0435) centre (-556.6728, 327.9457) ccw projected
  line L117 (-556.6728, 307.848) -> (-573.6273, 307.848) projected
  arc A148 (-573.6273, 394.589) -> (-573.6273, 354.3935) centre (-573.6273, 374.4912) ccw projected
  line L118 (-573.6273, 394.589) -> (-556.6728, 394.589) projected
  arc A149 (-556.6728, 354.3935) -> (-556.6728, 394.589) centre (-556.6728, 374.4912) ccw projected
  line L119 (-556.6728, 354.3935) -> (-573.6273, 354.3935) projected
  arc A150 (-573.6273, 441.1345) -> (-573.6273, 400.939) centre (-573.6273, 421.0367) ccw projected
  line L120 (-573.6273, 441.1345) -> (-556.6728, 441.1345) projected
  arc A151 (-556.6728, 400.939) -> (-556.6728, 441.1345) centre (-556.6728, 421.0367) ccw projected
  line L121 (-556.6728, 400.939) -> (-573.6273, 400.939) projected
  arc A152 (-573.6273, 487.68) -> (-573.6273, 447.4845) centre (-573.6273, 467.5822) ccw projected
  line L122 (-573.6273, 487.68) -> (-556.6728, 487.68) projected
  arc A153 (-556.6728, 447.4845) -> (-556.6728, 487.68) centre (-556.6728, 467.5822) ccw projected
  line L123 (-556.6728, 447.4845) -> (-573.6273, 447.4845) projected
  arc A154 (-637.1272, 68.7705) -> (-637.1272, 28.575) centre (-637.1272, 48.6727) ccw projected
  line L124 (-637.1272, 68.7705) -> (-620.1728, 68.7705) projected
  arc A155 (-620.1728, 28.575) -> (-620.1728, 68.7705) centre (-620.1728, 48.6727) ccw projected
  line L125 (-620.1728, 28.575) -> (-637.1272, 28.575) projected
  arc A156 (-637.1273, 115.316) -> (-637.1273, 75.1205) centre (-637.1273, 95.2182) ccw projected
  line L126 (-637.1273, 115.316) -> (-620.1728, 115.316) projected
  arc A157 (-620.1728, 75.1205) -> (-620.1728, 115.316) centre (-620.1728, 95.2182) ccw projected
  line L127 (-620.1728, 75.1205) -> (-637.1273, 75.1205) projected
  arc A158 (-637.1273, 161.8615) -> (-637.1273, 121.666) centre (-637.1273, 141.7637) ccw projected
  line L128 (-637.1273, 161.8615) -> (-620.1728, 161.8615) projected
  arc A159 (-620.1728, 121.666) -> (-620.1728, 161.8615) centre (-620.1728, 141.7637) ccw projected
  line L129 (-620.1728, 121.666) -> (-637.1273, 121.666) projected
  arc A160 (-637.1273, 208.407) -> (-637.1273, 168.2115) centre (-637.1273, 188.3092) ccw projected
  line L130 (-637.1273, 208.407) -> (-620.1728, 208.407) projected
  arc A161 (-620.1728, 168.2115) -> (-620.1728, 208.407) centre (-620.1728, 188.3092) ccw projected
  line L131 (-620.1728, 168.2115) -> (-637.1273, 168.2115) projected
  arc A162 (-637.1273, 254.9525) -> (-637.1273, 214.757) centre (-637.1273, 234.8547) ccw projected
  line L132 (-637.1273, 254.9525) -> (-620.1728, 254.9525) projected
  arc A163 (-620.1728, 214.757) -> (-620.1728, 254.9525) centre (-620.1728, 234.8547) ccw projected
  line L133 (-620.1728, 214.757) -> (-637.1273, 214.757) projected
  arc A164 (-637.1273, 301.498) -> (-637.1273, 261.3025) centre (-637.1273, 281.4002) ccw projected
  line L134 (-637.1273, 301.498) -> (-620.1728, 301.498) projected
  arc A165 (-620.1728, 261.3025) -> (-620.1728, 301.498) centre (-620.1728, 281.4002) ccw projected
  line L135 (-620.1728, 261.3025) -> (-637.1273, 261.3025) projected
  arc A166 (-637.1273, 348.0435) -> (-637.1273, 307.848) centre (-637.1273, 327.9457) ccw projected
  line L136 (-637.1273, 348.0435) -> (-620.1728, 348.0435) projected
  arc A167 (-620.1728, 307.848) -> (-620.1728, 348.0435) centre (-620.1728, 327.9457) ccw projected
  line L137 (-620.1728, 307.848) -> (-637.1273, 307.848) projected
  arc A168 (-637.1273, 394.589) -> (-637.1273, 354.3935) centre (-637.1273, 374.4912) ccw projected
  line L138 (-637.1273, 394.589) -> (-620.1728, 394.589) projected
  arc A169 (-620.1728, 354.3935) -> (-620.1728, 394.589) centre (-620.1728, 374.4912) ccw projected
  line L139 (-620.1728, 354.3935) -> (-637.1273, 354.3935) projected
  arc A170 (-637.1273, 441.1345) -> (-637.1273, 400.939) centre (-637.1273, 421.0367) ccw projected
  line L140 (-637.1273, 441.1345) -> (-620.1728, 441.1345) projected
  arc A171 (-620.1728, 400.939) -> (-620.1728, 441.1345) centre (-620.1728, 421.0367) ccw projected
  line L141 (-620.1728, 400.939) -> (-637.1273, 400.939) projected
  arc A172 (-637.1273, 487.68) -> (-637.1273, 447.4845) centre (-637.1273, 467.5822) ccw projected
  line L142 (-637.1273, 487.68) -> (-620.1728, 487.68) projected
  arc A173 (-620.1728, 447.4845) -> (-620.1728, 487.68) centre (-620.1728, 467.5822) ccw projected
  line L143 (-620.1728, 447.4845) -> (-637.1273, 447.4845) projected
  circle A174 centre (-12.7, 503.555) radius 2.0828 projected
  circle A175 centre (-12.7, 12.7) radius 2.0828 projected
  circle A176 centre (-38.1, 503.555) radius 2.0828 projected
  circle A177 centre (-38.1, 12.7) radius 2.0828 projected
  circle A178 centre (-63.5, 503.555) radius 2.0828 projected
  circle A179 centre (-63.5, 12.7) radius 2.0828 projected
  circle A180 centre (-88.9, 503.555) radius 2.0828 projected
  circle A181 centre (-88.9, 12.7) radius 2.0828 projected
  circle A182 centre (-114.3, 503.555) radius 2.0828 projected
  circle A183 centre (-114.3, 12.7) radius 2.0828 projected
  circle A184 centre (-139.7, 503.555) radius 2.0828 projected
  circle A185 centre (-139.7, 12.7) radius 2.0828 projected
  circle A186 centre (-165.1, 503.555) radius 2.0828 projected
  circle A187 centre (-165.1, 12.7) radius 2.0828 projected
  circle A188 centre (-190.5, 503.555) radius 2.0828 projected
  circle A189 centre (-190.5, 12.7) radius 2.0828 projected
  circle A190 centre (-215.9, 503.555) radius 2.0828 projected
  circle A191 centre (-215.9, 12.7) radius 2.0828 projected
  circle A192 centre (-241.3, 503.555) radius 2.0828 projected
  circle A193 centre (-241.3, 12.7) radius 2.0828 projected
  circle A194 centre (-266.7, 503.555) radius 2.0828 projected
  circle A195 centre (-266.7, 12.7) radius 2.0828 projected
  circle A196 centre (-292.1, 503.555) radius 2.0828 projected
  circle A197 centre (-292.1, 12.7) radius 2.0828 projected
  circle A198 centre (-317.5, 503.555) radius 2.0828 projected
  circle A199 centre (-317.5, 12.7) radius 2.0828 projected
  circle A200 centre (-342.9, 503.555) radius 2.0828 projected
  circle A201 centre (-342.9, 12.7) radius 2.0828 projected
  circle A202 centre (-368.3, 503.555) radius 2.0828 projected
  circle A203 centre (-368.3, 12.7) radius 2.0828 projected
  circle A204 centre (-393.7, 503.555) radius 2.0828 projected
  circle A205 centre (-393.7, 12.7) radius 2.0828 projected
  circle A206 centre (-419.1, 503.555) radius 2.0828 projected
  circle A207 centre (-419.1, 12.7) radius 2.0828 projected
  circle A208 centre (-444.5, 503.555) radius 2.0828 projected
  circle A209 centre (-444.5, 12.7) radius 2.0828 projected
  circle A210 centre (-469.9, 503.555) radius 2.0828 projected
  circle A211 centre (-469.9, 12.7) radius 2.0828 projected
  circle A212 centre (-495.3, 503.555) radius 2.0828 projected
  circle A213 centre (-495.3, 12.7) radius 2.0828 projected
  circle A214 centre (-520.7, 503.555) radius 2.0828 projected
  circle A215 centre (-520.7, 12.7) radius 2.0828 projected
  circle A216 centre (-546.1, 503.555) radius 2.0828 projected
  circle A217 centre (-546.1, 12.7) radius 2.0828 projected
  circle A218 centre (-571.5, 503.555) radius 2.0828 projected
  circle A219 centre (-571.5, 12.7) radius 2.0828 projected
  circle A220 centre (-596.9, 503.555) radius 2.0828 projected
  circle A221 centre (-596.9, 12.7) radius 2.0828 projected
  circle A222 centre (-622.3, 503.555) radius 2.0828 projected
  circle A223 centre (-622.3, 12.7) radius 2.0828 projected
  circle A224 centre (-647.7, 503.555) radius 2.0828 projected
  circle A225 centre (-647.7, 12.7) radius 2.0828 projected
  circle A226 centre (-673.1, 503.555) radius 2.0828 projected
  circle A227 centre (-673.1, 12.7) radius 2.0828 projected
  line L144 (-685.8, 0) -> (-685.8, 516.255) projected
  line L145 (0, 0) -> (-685.8, 0) projected
  line L146 (0, 516.255) -> (0, 0) projected
  line L147 (-685.8, 516.255) -> (0, 516.255) projected